Autodesk Fusion 360 part; units mm, degrees
(part 3 of 5)
  spline S405 degree 3 poles (17.0095, -37.7346) (17.0401, -37.6962) (17.0716, -37.6554) (17.1042, -37.6133) knots 24 24 24 24 25 25 25 25
  spline S406 degree 3 poles (17.1042, -37.6133) (17.3273, -37.3244) (17.6051, -36.9649) (17.951, -36.9312) knots 25 25 25 25 26 26 26 26
  spline S407 degree 3 poles (17.951, -36.9312) (18.1537, -36.9124) (18.4001, -37.0615) (18.43, -37.2905) knots 26 26 26 26 27 27 27 27
  ellipse E60 centre (17.4573, -38.1763) end of major axis (17.2727, -40.3787) minor radius 0.995 (18.3658, -38.8335) -> (18.43, -37.2905) ccw
  spline S408 degree 3 poles (18.3658, -38.8335) (18.1975, -39.648) (17.7584, -40.4986) (17.161, -41.1673) knots 28 28 28 28 29 29 29 29
  spline S409 degree 3 poles (9.1607, -35.1495) (9.5148, -36.3147) (10.6476, -37.0396) (11.7092, -37.5945) (11.9284, -37.7091) (12.1669, -37.8283) (12.4344, -37.9569) knots 0 0 0 0 1 1 1 2 2 2 2
  spline S410 degree 3 poles (12.4344, -37.9569) (12.4326, -37.9612) (12.4318, -37.9657) (12.4301, -37.97) knots 2 2 2 2 3 3 3 3
  spline S411 degree 3 poles (12.4301, -37.97) (12.403, -38.0389) (12.3786, -38.1093) (12.3605, -38.1829) knots 3 3 3 3 4 4 4 4
  spline S412 degree 3 poles (12.3605, -38.1829) (12.3365, -38.2818) (12.3232, -38.3821) (12.3214, -38.481) (12.3137, -38.8856) (12.6908, -39.1663) (12.9935, -39.3921) (13.0593, -39.4412) (13.1224, -39.4879) (13.1768, -39.533) knots 4 4 4 4 5 5 5 6 6 6 7 7 7 7
  spline S413 degree 3 poles (13.1768, -39.533) (13.3089, -39.6428) (13.4471, -39.7455) (13.5806, -39.8449) knots 7 7 7 7 8 8 8 8
  line L61 (13.5806, -39.8449) -> (13.6872, -39.9245)
  spline S414 degree 3 poles (13.6872, -39.9245) (14.0165, -40.1718) (14.3068, -40.4614) (14.5874, -40.7415) (14.8134, -40.9671) (15.0471, -41.2003) (15.304, -41.4155) knots 9 9 9 9 10 10 10 11 11 11 11
  spline S415 degree 3 poles (15.304, -41.4155) (15.3519, -41.4555) (15.3989, -41.4971) (15.4457, -41.5385) knots 11 11 11 11 12 12 12 12
  spline S416 degree 3 poles (15.4457, -41.5385) (15.6965, -41.7603) (15.9561, -41.9898) (16.3325, -42.0079) knots 12 12 12 12 13 13 13 13
  spline S417 degree 3 poles (16.3325, -42.0079) (16.3909, -42.0107) (16.4474, -42.0082) (16.5021, -42.0011) (16.5782, -41.9911) (16.6497, -41.9697) (16.7191, -41.9437) (16.7888, -41.9176) (16.8557, -41.8855) (16.9193, -41.8469) (17.1111, -41.7304) (17.2772, -41.5666) (17.4241, -41.4024) knots 13 13 13 13 14 14 14 15 15 15 16 16 16 17 17 17 17
  spline S418 degree 3 poles (17.4241, -41.4024) (17.4279, -41.3981) (17.4313, -41.3935) (17.4351, -41.3892) (17.5055, -41.3099) (17.5736, -41.2281) (17.6397, -41.1443) (17.6657, -41.1113) (17.69, -41.0771) (17.7154, -41.0435) (17.7581, -40.9868) (17.8006, -40.9299) (17.8412, -40.8716) (17.8689, -40.8318) (17.8953, -40.7912) (17.922, -40.7507) knots 17 17 17 17 18 18 18 19 19 19 20 20 20 21 21 21 22 22 22 22
  spline S419 degree 3 poles (17.922, -40.7507) (17.9589, -40.6947) (17.9954, -40.6385) (18.0304, -40.5813) (18.0545, -40.5418) (18.0778, -40.5022) (18.1009, -40.4622) knots 22 22 22 22 23 23 23 24 24 24 24
  spline S420 degree 3 poles (18.1009, -40.4622) (18.1188, -40.4315) (18.1381, -40.4015) (18.1553, -40.3705) knots 24 24 24 24 25 25 25 25
  spline S421 degree 3 poles (18.1553, -40.3705) (18.6984, -40.5996) (19.175, -40.8092) (19.6083, -41.0094) knots 25 25 25 25 26 26 26 26
  spline S422 degree 3 poles (19.6083, -41.0094) (19.9314, -41.2063) (20.2654, -41.4182) (20.629, -41.6572) knots 26 26 26 26 27 27 27 27
  spline S423 degree 3 poles (20.629, -41.6572) (20.7153, -41.7141) (20.8008, -41.7723) (20.8862, -41.8305) knots 27 27 27 27 28 28 28 28
  line L62 (20.8862, -41.8305) -> (21.1231, -41.9905)
  spline S424 degree 3 poles (21.1231, -41.9905) (21.2965, -42.1069) (21.47, -42.2232) (21.6414, -42.3417) (21.7547, -42.4201) (21.8669, -42.4995) (21.9792, -42.579) knots 29 29 29 29 30 30 30 31 31 31 31
  line L63 (21.9792, -42.579) -> (22.2476, -42.7678)
  spline S425 degree 3 poles (22.2476, -42.7678) (22.3833, -42.8629) (22.5192, -42.9581) (22.6541, -43.054) knots 32 32 32 32 33 33 33 33
  line L64 (22.6541, -43.054) -> (23.3329, -43.5393)
  spline S426 degree 3 poles (23.3329, -43.5393) (23.3275, -43.557) (23.3242, -43.5743) (23.3195, -43.5919) knots 34 34 34 34 35 35 35 35
  spline S427 degree 3 poles (23.3195, -43.5919) (23.3148, -43.6089) (23.3104, -43.6257) (23.3065, -43.6426) knots 35 35 35 35 36 36 36 36
  spline S428 degree 3 poles (23.3065, -43.6426) (23.2921, -43.7038) (23.2805, -43.7645) (23.2748, -43.8235) knots 36 36 36 36 37 37 37 37
  spline S429 degree 3 poles (23.2748, -43.8235) (23.2748, -43.8237) (23.2747, -43.8239) (23.2747, -43.824) knots 37 37 37 37 38 38 38 38
  spline S430 degree 3 poles (23.2747, -43.824) (23.253, -44.048) (23.3387, -44.3191) (23.3843, -44.4441) knots 38 38 38 38 39 39 39 39
  ellipse E61 centre (23.3854, -44.4319) end of major axis (23.3496, -44.3317) minor radius 0.0052 (23.3843, -44.4441) -> (23.401, -44.4882) ccw
  spline S431 degree 3 poles (23.401, -44.4882) (23.4621, -44.6444) (23.5572, -44.7939) (23.7005, -44.9589) knots 40 40 40 40 41 41 41 41
  spline S432 degree 3 poles (23.7005, -44.9589) (23.9176, -45.2076) (24.135, -45.3973) (24.3661, -45.5393) knots 41 41 41 41 42 42 42 42
  line L65 (24.3661, -45.5393) -> (24.4057, -45.5638)
  spline S433 degree 3 poles (24.4057, -45.5638) (24.4421, -45.5865) (24.4789, -45.6094) (24.5162, -45.6294) knots 43 43 43 43 44 44 44 44
  arc A9 (24.5162, -45.6294) -> (24.5477, -45.6426) centre (24.6008, -45.4712) ccw
  spline S434 degree 3 poles (24.5477, -45.6426) (24.6194, -45.6647) (24.6914, -45.6848) (24.7636, -45.7029) (24.7855, -45.7084) (24.8076, -45.7126) (24.8296, -45.7178) (24.8802, -45.7297) (24.9309, -45.7417) (24.9818, -45.7516) (25.0059, -45.7563) (25.03, -45.7597) (25.0541, -45.764) (25.1033, -45.7727) (25.1525, -45.7815) (25.2018, -45.7884) (25.2258, -45.7918) (25.2499, -45.794) (25.274, -45.7969) (25.3237, -45.803) (25.3734, -45.8091) (25.4232, -45.8133) (25.4471, -45.8154) (25.471, -45.8163) (25.495, -45.818) (25.545, -45.8213) (25.595, -45.8247) (25.6451, -45.8262) (25.6699, -45.827) (25.6947, -45.8268) (25.7195, -45.8271) (25.7686, -45.8277) (25.8176, -45.8283) (25.8668, -45.8272) (25.8941, -45.8266) (25.9213, -45.825) (25.9486, -45.8238) (25.9947, -45.8219) (26.0408, -45.8199) (26.0869, -45.8165) (26.1189, -45.8141) (26.1509, -45.8106) (26.1829, -45.8075) knots 45 45 45 45 46 46 46 47 47 47 48 48 48 49 49 49 50 50 50 51 51 51 52 52 52 53 53 53 54 54 54 55 55 55 56 56 56 57 57 57 58 58 58 59 59 59 59
  spline S435 degree 3 poles (26.1829, -45.8075) (26.2128, -45.8045) (26.2427, -45.8027) (26.2726, -45.7991) knots 59 59 59 59 60 60 60 60
  spline S436 degree 3 poles (26.2726, -45.7991) (27.1902, -46.394) (27.959, -46.9051) (28.7109, -47.4517) knots 60 60 60 60 61 61 61 61
  line L66 (28.7109, -47.4517) -> (28.9558, -47.6293)
  spline S437 degree 3 poles (28.9558, -47.6293) (29.1234, -47.7506) (29.2998, -47.8781) (29.4804, -48.0117) knots 62 62 62 62 63 63 63 63
  line L67 (29.4804, -48.0117) -> (29.484, -48.0146)
  line L68 (29.484, -48.0146) -> (30.5036, -48.8221)
  line L69 (30.5036, -48.8221) -> (30.5435, -48.8589)
  spline S438 degree 3 poles (30.5435, -48.8589) (30.7296, -49.0293) (31.5071, -49.7424) (32.403, -50.5655) knots 66 66 66 66 67 67 67 67
  spline S439 degree 3 poles (32.403, -50.5655) (32.3945, -50.5754) (32.3858, -50.5865) (32.3773, -50.5966) knots 67 67 67 67 68 68 68 68
  spline S440 degree 3 poles (32.3773, -50.5966) (32.371, -50.6041) (32.3648, -50.6117) (32.3586, -50.6192) knots 68 68 68 68 69 69 69 69
  spline S441 degree 3 poles (32.3586, -50.6192) (32.3317, -50.6517) (32.3053, -50.6846) (32.2797, -50.718) knots 69 69 69 69 70 70 70 70
  spline S442 degree 3 poles (32.2797, -50.718) (32.2765, -50.7221) (32.2735, -50.7263) (32.2703, -50.7305) knots 70 70 70 70 71 71 71 71
  spline S443 degree 3 poles (32.2703, -50.7305) (32.243, -50.7665) (32.2164, -50.8029) (32.1908, -50.8399) knots 71 71 71 71 72 72 72 72
  spline S444 degree 3 poles (32.1908, -50.8399) (32.1886, -50.8431) (32.1865, -50.8465) (32.1842, -50.8497) knots 72 72 72 72 73 73 73 73
  ellipse E62 centre (32.7413, -51.7007) end of major axis (33.3078, -50.2436) minor radius 0.8939 (32.1842, -50.8497) -> (32.0918, -50.9957) ccw
  ellipse E63 centre (37.7927, -51.9009) end of major axis (31.806, -52.0345) minor radius 3.2559 (32.0918, -50.9957) -> (32.0102, -51.1478) ccw
  spline S445 degree 3 poles (32.0102, -51.1478) (31.9954, -51.1779) (31.9808, -51.208) (31.9676, -51.2388) (31.9597, -51.2571) (31.953, -51.2759) (31.9457, -51.2944) (31.9324, -51.3284) (31.9199, -51.3626) (31.9087, -51.3973) knots 75 75 75 75 76 76 76 77 77 77 78 78 78 78
  spline S446 degree 3 poles (31.9087, -51.3973) (31.9028, -51.4156) (31.8973, -51.4341) (31.892, -51.4526) knots 78 78 78 78 79 79 79 79
  spline S447 degree 3 poles (31.892, -51.4526) (31.8812, -51.4905) (31.8719, -51.529) (31.8638, -51.5678) (31.8602, -51.5846) (31.8563, -51.6013) (31.8533, -51.6182) (31.8434, -51.6744) (31.8357, -51.7313) (31.832, -51.7894) (31.8262, -51.8814) (31.8306, -51.9755) (31.8454, -52.0693) knots 79 79 79 79 80 80 80 81 81 81 82 82 82 83 83 83 83
  spline S448 degree 3 poles (31.8454, -52.0693) (31.9055, -52.4449) (32.2971, -52.6397) (32.6118, -52.7963) knots 83 83 83 83 84 84 84 84
  spline S449 degree 3 poles (32.6118, -52.7963) (32.679, -52.8298) (32.7434, -52.8616) (32.7995, -52.8933) (32.9337, -52.9691) (33.072, -53.038) (33.2059, -53.1047) knots 84 84 84 84 85 85 85 86 86 86 86
  line L70 (33.2059, -53.1047) -> (33.3265, -53.165)
  spline S450 degree 3 poles (33.3265, -53.165) (33.6649, -53.3349) (33.9612, -53.5403) (34.2749, -53.7577) (34.5167, -53.9253) (34.7667, -54.0984) (35.0351, -54.2517) knots 87 87 87 87 88 88 88 89 89 89 89
  spline S451 degree 3 poles (35.0351, -54.2517) (35.0845, -54.2801) (35.1336, -54.3099) (35.1825, -54.3397) (35.425, -54.4873) (35.699, -54.6519) (36.0293, -54.6249) knots 89 89 89 89 90 90 90 91 91 91 91
  spline S452 degree 3 poles (36.0293, -54.6249) (36.0435, -54.6237) (36.0573, -54.6244) (36.0717, -54.6225) knots 91 91 91 91 92 92 92 92
  spline S453 degree 3 poles (36.0717, -54.6225) (36.1197, -54.6162) (36.1664, -54.6051) (36.2123, -54.5912) knots 92 92 92 92 93 93 93 93
  spline S454 degree 3 poles (36.2123, -54.5912) (36.2304, -54.5858) (36.2474, -54.5786) (36.2649, -54.5721) knots 93 93 93 93 94 94 94 94
  spline S455 degree 3 poles (36.2649, -54.5721) (36.2903, -54.5626) (36.3154, -54.5527) (36.3395, -54.5412) (36.3627, -54.5302) (36.3849, -54.5178) (36.4069, -54.5051) (36.4231, -54.4957) (36.4391, -54.486) (36.4547, -54.4758) (36.4817, -54.4581) (36.5078, -54.4393) (36.5331, -54.4192) (36.5377, -54.4156) (36.5425, -54.4129) (36.5471, -54.4092) knots 94 94 94 94 95 95 95 96 96 96 97 97 97 98 98 98 99 99 99 99
  spline S456 degree 3 poles (36.5471, -54.4092) (38.0743, -55.8341) (39.6611, -57.2394) (41.1968, -58.5994) (41.594, -58.9511) (41.991, -59.3028) (42.3876, -59.6551) (43.3096, -60.4743) (44.2328, -61.2921) (45.1561, -62.1099) knots 99 99 99 99 100 100 100 101 101 101 102 102 102 102
  line L71 (45.1561, -62.1099) -> (46.4361, -63.2436)
  spline S457 degree 3 poles (46.4361, -63.2436) (46.6035, -63.4107) (46.7725, -63.5762) (46.9415, -63.7418) (47.5199, -64.3084) (48.118, -64.8943) (48.6322, -65.5327) (48.7961, -65.7362) (48.9498, -65.957) (49.0985, -66.1706) (49.2301, -66.3596) (49.3662, -66.5551) (49.5114, -66.7419) (49.5584, -66.8024) (49.6059, -66.8628) (49.6535, -66.9231) knots 103 103 103 103 104 104 104 105 105 105 106 106 106 107 107 107 108 108 108 108
  spline S458 degree 3 poles (49.6535, -66.9231) (49.2873, -66.8806) (48.8648, -66.8491) (48.4098, -66.8491) (47.5059, -66.8491) (46.48, -66.9735) (45.5423, -67.3771) (45.5269, -67.3837) (45.5116, -67.391) (45.4962, -67.3978) (45.4063, -67.4375) (45.3174, -67.48) (45.2294, -67.525) (45.2042, -67.538) (45.1789, -67.5506) (45.1538, -67.564) (45.053, -67.6178) (44.9531, -67.6743) (44.8555, -67.7358) knots 108 108 108 108 109 109 109 110 110 110 111 111 111 112 112 112 113 113 113 114 114 114 114
  spline S459 degree 3 poles (44.8555, -67.7358) (44.844, -67.7431) (44.8329, -67.7513) (44.8215, -67.7587) knots 114 114 114 114 115 115 115 115
  spline S460 degree 3 poles (44.8215, -67.7587) (44.7364, -67.8132) (44.6531, -67.8713) (44.571, -67.9321) (44.5417, -67.9538) (44.5127, -67.9763) (44.4838, -67.9988) (44.457, -68.0197) (44.4294, -68.0391) (44.403, -68.0607) (44.3635, -68.0929) (44.3268, -68.1276) (44.2887, -68.1611) (44.2679, -68.1793) (44.2459, -68.1951) (44.2254, -68.2138) (44.2149, -68.2233) (44.2054, -68.2337) (44.1951, -68.2433) knots 115 115 115 115 116 116 116 117 117 117 118 118 118 119 119 119 120 120 120 121 121 121 121
  spline S461 degree 3 poles (44.1951, -68.2433) (44.1623, -68.2738) (44.131, -68.3055) (44.0993, -68.3369) (44.059, -68.3767) (44.0187, -68.4166) (43.9801, -68.458) (43.9482, -68.4921) (43.9176, -68.5275) (43.8868, -68.5627) (43.8511, -68.6035) (43.8155, -68.6446) (43.7813, -68.6868) (43.7505, -68.7248) (43.7209, -68.7639) (43.6914, -68.803) (43.6598, -68.8448) (43.6285, -68.8868) (43.5984, -68.9299) (43.5691, -68.9717) (43.5408, -69.0145) (43.5129, -69.0575) (43.4852, -69.1002) (43.4579, -69.1432) (43.4314, -69.1871) (43.404, -69.2327) (43.3774, -69.279) (43.3513, -69.3259) (43.327, -69.3696) (43.3033, -69.4138) (43.2802, -69.4587) knots 121 121 121 121 122 122 122 123 123 123 124 124 124 125 125 125 126 126 126 127 127 127 128 128 128 129 129 129 130 130 130 131 131 131 131
  arc A10 (43.2802, -69.4587) -> (43.2065, -69.608) centre (47.6087, -71.6871) ccw
  spline S462 degree 3 poles (43.2065, -69.608) (43.1852, -69.6531) (43.1646, -69.6988) (43.1445, -69.7449) (43.1217, -69.7972) (43.0995, -69.85) (43.0782, -69.9036) (43.0596, -69.9504) (43.042, -69.998) (43.0246, -70.0458) (43.0045, -70.101) (42.9847, -70.1566) (42.9661, -70.2133) knots 132 132 132 132 133 133 133 134 134 134 135 135 135 136 136 136 136
  spline S463 degree 3 poles (42.9661, -70.2133) (42.9502, -70.2619) (42.9353, -70.3115) (42.9205, -70.3611) (42.9032, -70.4191) (42.886, -70.4772) (42.8703, -70.5365) knots 136 136 136 136 137 137 137 138 138 138 138
  spline S464 degree 3 poles (42.8703, -70.5365) (42.8567, -70.5875) (42.8444, -70.6397) (42.832, -70.6917) (42.8177, -70.7519) (42.8033, -70.812) (42.7905, -70.8735) (42.7793, -70.9275) (42.7696, -70.9827) (42.7595, -71.0377) (42.7482, -71.0995) (42.7366, -71.161) (42.7269, -71.2241) (42.7179, -71.282) (42.7106, -71.3414) (42.7029, -71.4004) (42.6947, -71.4629) (42.686, -71.5249) (42.6793, -71.5886) (42.6726, -71.6514) (42.6678, -71.7159) (42.6625, -71.7799) (42.6574, -71.8422) (42.6515, -71.9038) (42.6476, -71.9672) (42.6434, -72.0371) (42.6414, -72.1088) (42.6387, -72.1799) knots 138 138 138 138 139 139 139 140 140 140 141 141 141 142 142 142 143 143 143 144 144 144 145 145 145 146 146 146 147 147 147 147
  spline S465 degree 3 poles (42.6387, -72.1799) (42.6365, -72.2398) (42.6332, -72.2987) (42.6321, -72.3596) (42.6305, -72.443) (42.6315, -72.5286) (42.6321, -72.6138) (42.6324, -72.6647) (42.6315, -72.7144) (42.6326, -72.766) (42.6355, -72.904) (42.6409, -73.0442) (42.6492, -73.1867) knots 147 147 147 147 148 148 148 149 149 149 150 150 150 151 151 151 151
  spline S466 degree 3 poles (42.6492, -73.1867) (42.6534, -73.2587) (42.7009, -73.3208) (42.7691, -73.3438) knots 151 151 151 151 152 152 152 152
  spline S467 degree 3 poles (42.7691, -73.3438) (42.783, -73.3484) (42.8274, -73.363) (42.8976, -73.3839) knots 152 152 152 152 153 153 153 153
  line L72 (42.8976, -73.3839) -> (42.8987, -73.3843)
  spline S468 degree 3 poles (42.8987, -73.3843) (42.9207, -73.3908) (42.9455, -73.3981) (42.9724, -73.4058) (42.9888, -73.4105) (43.0076, -73.4156) (43.0258, -73.4207) (43.0383, -73.4242) (43.0498, -73.4275) (43.0631, -73.4311) (43.0897, -73.4384) (43.1189, -73.4461) (43.1487, -73.4539) (43.1558, -73.4557) (43.1623, -73.4575) (43.1695, -73.4594) knots 154 154 154 154 155 155 155 156 156 156 157 157 157 158 158 158 159 159 159 159
  spline S469 degree 3 poles (43.1695, -73.4594) (43.2046, -73.4684) (43.2421, -73.4778) (43.2811, -73.4874) knots 159 159 159 159 160 160 160 160
  line L73 (43.2811, -73.4874) -> (43.2902, -73.4897)
  spline S470 degree 3 poles (43.2902, -73.4897) (43.3326, -73.5) (43.3774, -73.5106) (43.4242, -73.5213) knots 161 161 161 161 162 162 162 162
  line L74 (43.4242, -73.5213) -> (43.4245, -73.5214)
  spline S471 degree 3 poles (43.4245, -73.5214) (44.4657, -73.76) (46.5503, -74.0551) (48.2956, -73.1753) knots 163 163 163 163 164 164 164 164
  line L75 (48.2956, -73.1753) -> (48.2962, -73.175)
  arc A11 (48.2962, -73.175) -> (48.5289, -73.0493) centre (46.1913, -69.0011) ccw
  spline S472 degree 3 poles (48.5289, -73.0493) (48.5315, -73.0478) (48.534, -73.0463) (48.5365, -73.0448) (48.6109, -73.0016) (48.6846, -72.9562) (48.7574, -72.9083) knots 166 166 166 166 167 167 167 168 168 168 168
  spline S473 degree 3 poles (48.7574, -72.9083) (48.759, -72.9072) (48.7607, -72.9063) (48.7624, -72.9052) knots 168 168 168 168 169 169 169 169
  spline S474 degree 3 poles (48.7624, -72.9052) (48.7659, -72.9029) (48.7691, -72.9003) (48.7726, -72.898) knots 169 169 169 169 170 170 170 170
  spline S475 degree 3 poles (48.7726, -72.898) (48.8213, -72.8656) (48.8703, -72.8341) (48.9181, -72.7996) (48.9366, -72.7863) (48.9535, -72.7713) (48.9717, -72.7577) (48.9923, -72.7423) (49.0121, -72.726) (49.0324, -72.7103) (49.2151, -72.5689) (49.3855, -72.414) (49.5439, -72.2456) (49.561, -72.2273) (49.5786, -72.2094) (49.5955, -72.1908) (49.6425, -72.139) (49.6881, -72.0856) (49.7329, -72.0314) (49.7503, -72.0104) (49.7674, -71.9892) (49.7844, -71.9679) (49.8293, -71.9115) (49.8734, -71.8542) (49.916, -71.7952) knots 170 170 170 170 171 171 171 172 172 172 173 173 173 174 174 174 175 175 175 176 176 176 177 177 177 178 178 178 178
  spline S476 degree 3 poles (49.916, -71.7952) (49.9278, -71.7789) (49.939, -71.7621) (49.9506, -71.7456) knots 178 178 178 178 179 179 179 179
  ellipse E64 centre (-485.3338, 431.1613) end of major axis (-1020.1941, 934.5888) minor radius 58.5616 (49.9506, -71.7456) -> (50.3479, -71.0732) ccw
  spline S477 degree 3 poles (50.3479, -71.0732) (50.3518, -71.0655) (50.3558, -71.058) (50.3596, -71.0503) (50.3952, -70.9771) (50.4288, -70.9019) (50.4618, -70.8259) knots 180 180 180 180 181 181 181 182 182 182 182
  spline S478 degree 3 poles (50.4618, -70.8259) (50.4714, -70.8038) (50.481, -70.7817) (50.4903, -70.7594) (50.5215, -70.685) (50.5514, -70.6095) (50.5801, -70.5324) (50.5884, -70.5099) (50.5964, -70.487) (50.6045, -70.4643) (50.7018, -70.1931) (50.7848, -69.9067) (50.8517, -69.6033) knots 182 182 182 182 183 183 183 184 184 184 185 185 185 186 186 186 186
  spline S479 degree 3 poles (50.8517, -69.6033) (50.8519, -69.6024) (50.8522, -69.6016) (50.8524, -69.6006) knots 186 186 186 186 187 187 187 187
  spline S480 degree 3 poles (50.8524, -69.6006) (50.871, -69.5159) (50.8876, -69.429) (50.9039, -69.3418) (50.9103, -69.3075) (50.917, -69.2733) (50.923, -69.2386) knots 187 187 187 187 188 188 188 189 189 189 189
  spline S481 degree 3 poles (50.923, -69.2386) (50.9374, -69.1559) (50.9506, -69.072) (50.9629, -68.9871) (50.9654, -68.9699) (50.9686, -68.9534) (50.971, -68.936) knots 189 189 189 189 190 190 190 191 191 191 191
  spline S482 degree 3 poles (50.971, -68.936) (51.0928, -69.1731) (51.2187, -69.4158) (51.3517, -69.6359) knots 191 191 191 191 192 192 192 192
  ellipse E65 centre (43.5345, -71.4342) end of major axis (50.5174, -82.0369) minor radius 7.7071 (52.4938, -72.6612) -> (51.3517, -69.6359) ccw
  spline S483 degree 3 poles (52.4938, -72.6612) (49.477, -76.0968) (48.1935, -79.0277) (48.6792, -81.3802) (49.1255, -83.5419) (50.9129, -84.3589) (50.9887, -84.3927) (51.0315, -84.4117) (51.0805, -84.4127) (51.1243, -84.3958) knots 193 193 193 193 194 194 194 195 195 195 196 196 196 196
  spline S484 degree 3 poles (51.1243, -84.3958) (51.2453, -84.3488) (51.3636, -84.2998) (51.4795, -84.2492) (51.5206, -84.2313) (51.5598, -84.2121) (51.6002, -84.1937) (51.6738, -84.1603) (51.7476, -84.1271) (51.819, -84.0922) (51.8665, -84.069) (51.9119, -84.0445) (51.9584, -84.0207) (52.0204, -83.989) (52.0828, -83.9576) (52.143, -83.9247) (52.1918, -83.8981) (52.2387, -83.8702) (52.2864, -83.8429) (52.3417, -83.8111) (52.3975, -83.7797) (52.4514, -83.7469) (52.4999, -83.7174) (52.5467, -83.6867) (52.5941, -83.6563) (52.6444, -83.6241) (52.6951, -83.592) (52.7441, -83.5588) (52.7912, -83.5269) (52.8366, -83.4939) (52.8825, -83.4612) (52.9293, -83.4277) (52.9764, -83.3943) (53.0219, -83.36) (53.0667, -83.3261) (53.1101, -83.2913) (53.1536, -83.2566) (53.1974, -83.2217) (53.2413, -83.1867) (53.2838, -83.1509) (53.3262, -83.1152) (53.3674, -83.0786) (53.4085, -83.042) (53.4496, -83.0054) (53.4907, -82.9687) (53.5305, -82.9312) (53.57, -82.894) (53.6085, -82.8561) (53.6467, -82.818) (53.6856, -82.7793) (53.7242, -82.7404) (53.7618, -82.7008) knots 196 196 196 196 197 197 197 198 198 198 199 199 199 200 200 200 201 201 201 202 202 202 203 203 203 204 204 204 205 205 205 206 206 206 207 207 207 208 208 208 209 209 209 210 210 210 211 211 211 212 212 212 213 213 213 213
  spline S485 degree 3 poles (53.7618, -82.7008) (53.7982, -82.6624) (53.8338, -82.6233) (53.869, -82.5841) knots 213 213 213 213 214 214 214 214
  spline S486 degree 3 poles (53.869, -82.5841) (53.9058, -82.5431) (53.942, -82.5018) (53.9773, -82.4599) (54.0107, -82.4204) (54.0434, -82.3804) (54.0755, -82.3401) (54.1102, -82.2966) (54.1441, -82.2527) (54.1773, -82.2083) (54.2075, -82.168) (54.2371, -82.1273) (54.2662, -82.0862) knots 214 214 214 214 215 215 215 216 216 216 217 217 217 218 218 218 218
  spline S487 degree 3 poles (54.2662, -82.0862) (54.2987, -82.04) (54.3304, -81.9931) (54.3615, -81.9459) (54.3884, -81.9051) (54.4151, -81.864) (54.4409, -81.8224) (54.4714, -81.773) (54.5008, -81.723) (54.5298, -81.6726) (54.5535, -81.6314) (54.5772, -81.5903) (54.5998, -81.5484) (54.6281, -81.4959) (54.6551, -81.4425) (54.6818, -81.389) knots 218 218 218 218 219 219 219 220 220 220 221 221 221 222 222 222 223 223 223 223
  spline S488 degree 3 poles (54.6818, -81.389) (54.7025, -81.3474) (54.7234, -81.306) (54.743, -81.2638) (54.7689, -81.2084) (54.7931, -81.152) (54.8172, -81.0955) (54.8352, -81.0534) (54.8534, -81.0115) (54.8704, -80.9688) (54.8763, -80.9541) (54.883, -80.94) (54.8888, -80.9252) (54.9113, -80.8671) (54.9312, -80.8084) (54.9518, -80.7498) (54.9582, -80.7315) (54.9657, -80.7138) (54.972, -80.6954) knots 223 223 223 223 224 224 224 225 225 225 226 226 226 227 227 227 228 228 228 229 229 229 229
  spline S489 degree 3 poles (54.972, -80.6954) (54.9733, -80.6915) (54.9743, -80.6875) (54.9756, -80.6835) knots 229 229 229 229 230 230 230 230
  arc A12 (54.9756, -80.6835) -> (55.0773, -80.3483) centre (49.3167, -78.7838) ccw
  spline S490 degree 3 poles (55.0773, -80.3483) (55.0809, -80.3349) (55.084, -80.3214) (55.0876, -80.308) knots 231 231 231 231 232 232 232 232
  spline S491 degree 3 poles (55.0876, -80.308) (55.1143, -80.2067) (55.1384, -80.105) (55.16, -80.0029) (55.1638, -79.985) (55.1676, -79.9671) (55.1712, -79.9492) knots 232 232 232 232 233 233 233 234 234 234 234
  ellipse E66 centre (24.4608, -64.2546) end of major axis (-5.574, -46.7642) minor radius 13.9771 (55.1712, -79.9492) -> (55.3003, -78.8826) ccw
  line L76 (55.3003, -78.8826) -> (55.301, -78.8667)
  ellipse E67 centre (37.5646, -70.719) end of major axis (20.8518, -59.3182) minor radius 10.5763 (55.301, -78.8667) -> (55.2771, -77.7932) ccw
  spline S492 degree 3 poles (55.2771, -77.7932) (55.2758, -77.7777) (55.2744, -77.7621) (55.273, -77.7466) (55.2641, -77.6466) (55.2536, -77.547) (55.2417, -77.4478) (55.2395, -77.429) (55.2375, -77.4101) (55.2352, -77.3914) knots 237 237 237 237 238 238 238 239 239 239 240 240 240 240
  spline S493 degree 3 poles (55.2352, -77.3914) (55.2216, -77.2828) (55.2063, -77.1748) (55.1894, -77.0674) (55.1833, -77.0284) (55.1762, -76.9898) (55.1696, -76.951) (55.1593, -76.89) (55.1488, -76.8292) (55.1376, -76.7687) (55.1254, -76.7034) (55.1126, -76.6386) (55.0995, -76.5739) (55.0944, -76.5491) (55.0892, -76.5244) (55.084, -76.4997) knots 240 240 240 240 241 241 241 242 242 242 243 243 243 244 244 244 245 245 245 245
  spline S494 degree 3 poles (55.084, -76.4997) (54.7762, -75.0337) (54.2156, -73.7332) (53.8123, -72.9225) knots 245 245 245 245 246 246 246 246
  ellipse E68 centre (48.0724, -66.8569) end of major axis (44.1035, -56.4654) minor radius 4.4389 (53.8123, -72.9225) -> (53.7916, -72.1467) ccw
  spline S495 degree 3 poles (53.7916, -72.1467) (54.1354, -72.7806) (54.5781, -73.438) (55.1292, -73.9842) knots 247 247 247 247 248 248 248 248
  spline S496 degree 3 poles (55.1292, -73.9842) (55.1337, -73.9886) (55.1382, -73.9931) (55.1426, -73.9975) (55.2006, -74.0546) (55.2599, -74.1101) (55.3202, -74.1645) (55.3349, -74.1777) (55.3493, -74.1911) (55.3641, -74.2041) knots 248 248 248 248 249 249 249 250 250 250 251 251 251 251
  spline S497 degree 3 poles (55.3641, -74.2041) (55.4151, -74.249) (55.4672, -74.2925) (55.5199, -74.3353) (55.5435, -74.3545) (55.5669, -74.3741) (55.5909, -74.3929) (55.6362, -74.4282) (55.6825, -74.462) (55.7289, -74.4957) (55.7605, -74.5186) (55.7918, -74.5419) (55.824, -74.564) (55.8646, -74.5919) (55.9064, -74.6181) (55.9479, -74.6446) (55.9865, -74.6691) (56.0246, -74.6942) (56.0639, -74.7176) (56.1013, -74.7397) (56.1398, -74.76) (56.1779, -74.7809) (56.2223, -74.8054) (56.2663, -74.8305) (56.3117, -74.8532) (56.3476, -74.8712) (56.3847, -74.8871) (56.4213, -74.904) (56.4698, -74.9265) (56.5178, -74.9498) (56.5675, -74.9703) (56.6066, -74.9864) (56.6472, -75) (56.687, -75.0149) (56.7351, -75.0328) (56.7826, -75.0519) (56.8318, -75.0679) knots 251 251 251 251 252 252 252 253 253 253 254 254 254 255 255 255 256 256 256 257 257 257 258 258 258 259 259 259 260 260 260 261 261 261 262 262 262 263 263 263 263
  spline S498 degree 3 poles (56.8318, -75.0679) (56.8333, -75.0684) (56.8347, -75.0691) (56.8363, -75.0696) knots 263 263 263 263 264 264 264 264
  spline S499 degree 3 poles (56.8363, -75.0696) (56.9029, -75.0912) (56.9702, -75.1087) (57.0375, -75.1263) knots 264 264 264 264 265 265 265 265
  spline S500 degree 3 poles (57.0375, -75.1263) (57.0601, -75.1321) (57.0818, -75.1398) (57.1045, -75.1452) knots 265 265 265 265 266 266 266 266
  line L77 (57.1045, -75.1452) -> (57.0886, -75.142)
  spline S501 degree 3 poles (57.0886, -75.142) (57.1061, -75.1462) (57.1239, -75.1487) (57.1415, -75.1527) (57.212, -75.1684) (57.2826, -75.1832) (57.3538, -75.1946) (57.3955, -75.2012) (57.4377, -75.205) (57.4796, -75.2101) (57.527, -75.2159) (57.5743, -75.2226) (57.6221, -75.2265) (57.6705, -75.2305) (57.7193, -75.2316) (57.768, -75.2336) (57.8099, -75.2353) (57.8517, -75.2378) (57.8939, -75.238) (57.9455, -75.2383) (57.9976, -75.236) (58.0496, -75.2341) (58.0894, -75.2327) (58.1291, -75.2318) (58.1691, -75.2291) (58.2229, -75.2254) (58.277, -75.2194) (58.3312, -75.2134) (58.3699, -75.2091) (58.4087, -75.2051) (58.4477, -75.1997) (58.5029, -75.1919) (58.5585, -75.1821) (58.6141, -75.172) (58.6526, -75.165) (58.6911, -75.1579) (58.7299, -75.1498) (58.7862, -75.1379) (58.8428, -75.1243) (58.8995, -75.11) (58.9381, -75.1002) (58.9767, -75.0902) (59.0155, -75.0794) (59.0724, -75.0634) (59.1295, -75.0461) (59.1869, -75.0278) (59.2263, -75.0151) (59.2658, -75.0019) (59.3054, -74.9881) (59.3623, -74.9683) (59.4195, -74.9475) (59.4767, -74.9253) (59.5174, -74.9096) (59.5583, -74.8929) (59.5992, -74.876) (59.6559, -74.8525) (59.7128, -74.8283) (59.7699, -74.8025) (59.8121, -74.7834) (59.8545, -74.7631) (59.8969, -74.7427) (59.953, -74.7158) (60.0092, -74.6886) (60.0657, -74.6595) (60.1102, -74.6365) (60.155, -74.6119) (60.1998, -74.5875) (60.2546, -74.5577) (60.3093, -74.5281) (60.3644, -74.4962) (60.4124, -74.4685) (60.4607, -74.4387) (60.5089, -74.4094) (60.5613, -74.3775) (60.6136, -74.3463) (60.6663, -74.3126) (60.7192, -74.2787) (60.7725, -74.2424) (60.8256, -74.2066) (60.8742, -74.174) (60.9227, -74.1424) (60.9715, -74.1082) (61.0339, -74.0645) (61.0966, -74.0179) (61.1593, -73.9717) (61.1995, -73.942) (61.2396, -73.9139) (61.28, -73.8832) (61.3835, -73.8045) (61.4874, -73.7228) (61.5919, -73.6373) (61.6301, -73.6059) (61.6529, -73.5606) (61.6561, -73.5128) (61.6572, -73.4968) (61.6562, -73.4805) (61.6528, -73.4644) knots 267 267 267 267 268 268 268 269 269 269 270 270 270 271 271 271 272 272 272 273 273 273 274 274 274 275 275 275 276 276 276 277 277 277 278 278 278 279 279 279 280 280 280 281 281 281 282 282 282 283 283 283 284 284 284 285 285 285 286 286 286 287 287 287 288 288 288 289 289 289 290 290 290 291 291 291 292 292 292 293 293 293 294 294 294 295 295 295 296 296 296 297 297 297 298 298 298 299 299 299 299
  spline S502 degree 3 poles (61.6528, -73.4644) (61.6517, -73.4595) (61.6491, -73.4476) (61.6454, -73.4317) knots 299 299 299 299 300 300 300 300
  spline S503 degree 3 poles (61.6454, -73.4317) (61.5771, -73.1385) (61.0291, -71.0534) (59.0331, -69.8622) (58.134, -69.3257) (57.0851, -69.0573) (55.8967, -69.0574) (55.119, -69.0575) (54.2811, -69.1737) (53.3867, -69.404) knots 300 300 300 300 301 301 301 302 302 302 303 303 303 303
  ellipse E69 centre (35.8916, -66.1831) end of major axis (20.5604, -52.0655) minor radius 13.7082 (53.3867, -69.404) -> (51.9599, -65.262) ccw
  spline S504 degree 3 poles (51.9599, -65.262) (53.2122, -65.7163) (54.5148, -65.9538) (55.6442, -66.1266) (56.138, -66.2022) (56.6543, -66.2661) (57.1538, -66.3279) (59.1045, -66.5694) (61.1217, -66.8191) (62.7538, -67.8227) knots 304 304 304 304 305 305 305 306 306 306 307 307 307 307
  spline S505 degree 3 poles (62.7538, -67.8227) (62.9133, -67.9429) (63.1017, -68.0812) (63.301, -68.2076) knots 307 307 307 307 308 308 308 308
  spline S506 degree 3 poles (63.301, -68.2076) (62.8168, -69.1853) (62.139, -71.0646) (62.6864, -73.1703) (62.7066, -73.2481) (62.7277, -73.326) (62.7514, -73.4044) (62.7584, -73.4278) (62.7665, -73.4513) (62.7739, -73.4747) knots 308 308 308 308 309 309 309 310 310 310 311 311 311 311
  spline S507 degree 3 poles (62.7739, -73.4747) (62.7967, -73.5469) (62.8205, -73.6191) (62.8463, -73.6917) (62.85, -73.702) (62.8529, -73.7122) (62.8566, -73.7226) knots 311 311 311 311 312 312 312 313 313 313 313
  spline S508 degree 3 poles (62.8566, -73.7226) (62.8622, -73.738) (62.8687, -73.7531) (62.8744, -73.7685) knots 313 313 313 313 314 314 314 314
  spline S509 degree 3 poles (62.8744, -73.7685) (62.8968, -73.8291) (62.9202, -73.8895) (62.9445, -73.9495) (62.9553, -73.9763) (62.9663, -74.003) (62.9775, -74.0296) (62.9868, -74.0518) (62.9952, -74.074) (63.0049, -74.0963) (63.0182, -74.1268) (63.033, -74.1568) (63.0468, -74.1871) knots 314 314 314 314 315 315 315 316 316 316 317 317 317 318 318 318 318
  spline S510 degree 3 poles (63.0468, -74.1871) (63.0643, -74.2259) (63.0819, -74.2647) (63.1003, -74.3032) (63.1206, -74.3459) (63.1419, -74.3883) (63.1632, -74.4306) knots 318 318 318 318 319 319 319 320 320 320 320
  spline S511 degree 3 poles (63.1632, -74.4306) (63.1861, -74.4762) (63.2091, -74.5218) (63.2332, -74.567) (63.2511, -74.6007) (63.27, -74.6341) (63.2885, -74.6677) knots 320 320 320 320 321 321 321 322 322 322 322
  spline S512 degree 3 poles (63.2885, -74.6677) (63.3177, -74.7203) (63.347, -74.7729) (63.3778, -74.8251) knots 322 322 322 322 323 323 323 323
  spline S513 degree 3 poles (63.3778, -74.8251) (63.3919, -74.8491) (63.4069, -74.8729) (63.4214, -74.8968) knots 323 323 323 323 324 324 324 324
  spline S514 degree 3 poles (63.4214, -74.8968) (63.4582, -74.9575) (63.4953, -75.018) (63.5342, -75.078) knots 324 324 324 324 325 325 325 325
  spline S515 degree 3 poles (63.5342, -75.078) (63.5424, -75.0906) (63.551, -75.103) (63.5592, -75.1155) knots 325 325 325 325 326 326 326 326
  ellipse E70 centre (232.856, -19.216) end of major axis (63.0285, -73.9056) minor radius 33.8867 (63.5592, -75.1155) -> (70.1202, -79.9149) ccw
  spline S516 degree 3 poles (70.1202, -79.9149) (70.1237, -79.9167) (70.1272, -79.9185) (70.1307, -79.9204) knots 327 327 327 327 328 328 328 328
  spline S517 degree 3 poles (70.1307, -79.9204) (70.2318, -79.9735) (70.3347, -80.026) (70.439, -80.0779) (70.4481, -80.0824) (70.4572, -80.087) (70.4663, -80.0915) knots 328 328 328 328 329 329 329 330 330 330 330
  spline S518 degree 3 poles (70.4663, -80.0915) (70.5646, -80.1446) (70.6644, -80.1971) (70.7656, -80.2491) (70.7795, -80.2562) (70.7934, -80.2633) (70.8074, -80.2704) (70.9045, -80.3199) (71.0028, -80.3689) (71.1026, -80.4174) (71.1225, -80.427) (71.1424, -80.4367) (71.1624, -80.4463) (71.2582, -80.4924) (71.355, -80.538) (71.4532, -80.5832) (71.4782, -80.5946) (71.5033, -80.606) (71.5284, -80.6175) (71.6231, -80.6605) (71.7187, -80.7032) (71.8156, -80.7453) (71.8462, -80.7587) (71.8771, -80.7719) (71.9079, -80.7851) (72.0011, -80.8251) (72.095, -80.8648) (72.1902, -80.904) (72.2266, -80.919) (72.2635, -80.9338) (72.3002, -80.9487) (72.3916, -80.9858) (72.4835, -81.0227) (72.5768, -81.059) (72.6196, -81.0757) (72.663, -81.0921) (72.7062, -81.1087) (72.7954, -81.1428) (72.8847, -81.1768) (72.9756, -81.2103) (73.0253, -81.2287) (73.076, -81.2467) (73.1262, -81.2649) (73.2125, -81.2961) (73.2988, -81.3272) (73.3866, -81.3579) (73.444, -81.3779) (73.5026, -81.3975) (73.5606, -81.4173) (73.6434, -81.4456) (73.7259, -81.4739) (73.8099, -81.5016) (73.8763, -81.5235) (73.944, -81.5449) (74.0111, -81.5665) (74.089, -81.5916) (74.1665, -81.6168) (74.2455, -81.6415) (74.3225, -81.6655) (74.4009, -81.6889) (74.4789, -81.7125) (74.5507, -81.7342) (74.6217, -81.7562) (74.6943, -81.7776) (74.7887, -81.8054) (74.8849, -81.8325) (74.9807, -81.8598) (75.0387, -81.8763) (75.0958, -81.8932) (75.1543, -81.9094) (75.3103, -81.9529) (75.468, -81.9956) (75.6278, -82.0375) knots 330 330 330 330 331 331 331 332 332 332 333 333 333 334 334 334 335 335 335 336 336 336 337 337 337 338 338 338 339 339 339 340 340 340 341 341 341 342 342 342 343 343 343 344 344 344 345 345 345 346 346 346 347 347 347 348 348 348 349 349 349 350 350 350 351 351 351 352 352 352 353 353 353 354 354 354 354
  spline S519 degree 3 poles (75.6278, -82.0375) (75.7152, -82.0579) (75.8006, -82.0123) (75.8331, -81.9307) knots 354 354 354 354 355 355 355 355
  spline S520 degree 3 poles (75.8331, -81.9307) (75.8476, -81.895) (75.923, -81.706) (76.0211, -81.3991) (76.0255, -81.3852) (76.0303, -81.3693) (76.0348, -81.355) knots 355 355 355 355 356 356 356 357 357 357 357
  spline S521 degree 3 poles (76.0348, -81.355) (76.0464, -81.3172) (76.0579, -81.2794) (76.07, -81.2383) knots 357 357 357 357 358 358 358 358
  spline S522 degree 3 poles (76.07, -81.2383) (76.08, -81.2044) (76.0903, -81.1673) (76.1005, -81.1313) knots 358 358 358 358 359 359 359 359
  spline S523 degree 3 poles (76.1005, -81.1313) (76.1076, -81.1068) (76.1146, -81.0838) (76.1218, -81.0585) (76.1362, -81.0079) (76.1508, -80.9541) (76.1654, -80.8998) (76.1689, -80.8869) (76.1724, -80.875) (76.1759, -80.8618) knots 359 359 359 359 360 360 360 361 361 361 362 362 362 362
  spline S524 degree 3 poles (76.1759, -80.8618) (76.1927, -80.7983) (76.2096, -80.7318) (76.2265, -80.6637) knots 362 362 362 362 363 363 363 363
  spline S525 degree 3 poles (76.2265, -80.6637) (76.2278, -80.6583) (76.2291, -80.6533) (76.2304, -80.6479) knots 363 363 363 363 364 364 364 364
  spline S526 degree 3 poles (76.2304, -80.6479) (76.5967, -79.8064) (77.0162, -78.5914) (77.1512, -77.2229) knots 364 364 364 364 365 365 365 365
  line L78 (77.1512, -77.2229) -> (72.1257, -81.7777)
  spline S527 degree 3 poles (72.1257, -81.7777) (72.1385, -81.6653) (72.1492, -81.5519) (72.1581, -81.4374) knots 366 366 366 366 367 367 367 367
  line L79 (72.1581, -81.4374) -> (72.6686, -75.3073)
  spline S528 degree 3 poles (72.6686, -75.3073) (72.6626, -75.1952) (72.6542, -75.0825) (72.6438, -74.9692) knots 368 368 368 368 369 369 369 369
  spline S529 degree 3 poles (72.6438, -74.9692) (72.6434, -74.9647) (72.6432, -74.9603) (72.6427, -74.9558) knots 369 369 369 369 370 370 370 370
  spline S530 degree 3 poles (72.6427, -74.9558) (72.6323, -74.8448) (72.6193, -74.7334) (72.6044, -74.6216) knots 370 370 370 370 371 371 371 371
  spline S531 degree 3 poles (72.6044, -74.6216) (72.6035, -74.6147) (72.6028, -74.608) (72.6018, -74.6012) knots 371 371 371 371 372 372 372 372
  spline S532 degree 3 poles (72.6018, -74.6012) (72.5869, -74.4921) (72.5692, -74.3828) (72.5497, -74.2732) knots 372 372 372 372 373 373 373 373
  spline S533 degree 3 poles (72.5497, -74.2732) (72.5479, -74.2634) (72.5465, -74.2536) (72.5447, -74.2438) knots 373 373 373 373 374 374 374 374
  spline S534 degree 3 poles (72.5447, -74.2438) (72.5251, -74.1369) (72.5027, -74.0297) (72.4784, -73.9225) knots 374 374 374 374 375 375 375 375
  spline S535 degree 3 poles (72.4784, -73.9225) (72.4757, -73.91) (72.4734, -73.8976) (72.4706, -73.8852) (72.4466, -73.7803) (72.4197, -73.6753) (72.391, -73.5703) (72.3869, -73.5555) (72.3835, -73.5406) (72.3793, -73.5258) (72.3508, -73.424) (72.3191, -73.3223) (72.2859, -73.2207) (72.2799, -73.2025) (72.2747, -73.1842) (72.2686, -73.1661) knots 375 375 375 375 376 376 376 377 377 377 378 378 378 379 379 379 380 380 380 380
  spline S536 degree 3 poles (72.2686, -73.1661) (72.2351, -73.0678) (72.1985, -72.9698) (72.1603, -72.8719) (72.1521, -72.8507) (72.1446, -72.8293) (72.1361, -72.8081) knots 380 380 380 380 381 381 381 382 382 382 382
  spline S537 degree 3 poles (72.1361, -72.8081) (72.0984, -72.7134) (72.0573, -72.619) (72.015, -72.5248) (72.0041, -72.5006) (71.9941, -72.4762) (71.9829, -72.452) (71.9407, -72.361) (71.8951, -72.2706) (71.8484, -72.1803) (71.8372, -72.1587) (71.8276, -72.1369) (71.8162, -72.1153) (71.8137, -72.1106) (71.8107, -72.1062) (71.8082, -72.1015) knots 382 382 382 382 383 383 383 384 384 384 385 385 385 386 386 386 387 387 387 387
  spline S538 degree 3 poles (71.8082, -72.1015) (71.7982, -72.0812) (71.7898, -72.0608) (71.7796, -72.0406) (71.7401, -71.9624) (71.6948, -71.8876) (71.6524, -71.8111) (71.6204, -71.7533) (71.59, -71.6946) (71.5564, -71.6377) (71.503, -71.5475) (71.445, -71.4599) (71.3874, -71.3721) (71.3506, -71.3159) (71.3149, -71.259) (71.2764, -71.2038) (71.2161, -71.1176) (71.1518, -71.0338) (71.0874, -70.9501) (71.0464, -70.8967) (71.0061, -70.8427) (70.9634, -70.7903) (70.896, -70.7077) (70.8249, -70.6274) (70.7534, -70.5473) (70.7084, -70.497) (70.664, -70.4463) (70.6174, -70.397) (70.5428, -70.318) (70.4648, -70.2411) (70.3861, -70.1647) (70.3373, -70.1174) (70.2887, -70.0699) (70.2384, -70.0236) (70.1565, -69.9483) (70.0715, -69.8749) (69.9854, -69.8021) (69.9331, -69.7579) (69.8807, -69.7138) (69.8268, -69.6706) (69.7374, -69.5989) (69.6453, -69.5289) (69.5516, -69.4598) (69.4958, -69.4187) (69.4397, -69.3778) (69.3824, -69.3376) (69.2856, -69.2697) (69.1864, -69.2033) (69.0853, -69.1381) (69.026, -69.0998) (68.9661, -69.062) (68.9052, -69.0246) (68.8012, -68.9607) (68.695, -68.898) (68.5865, -68.8368) (68.5236, -68.8013) (68.4598, -68.7664) (68.3954, -68.7318) (68.284, -68.6719) (68.1709, -68.613) (68.0552, -68.5559) (67.9887, -68.5231) (67.921, -68.4911) (67.8531, -68.4591) (67.7346, -68.4034) (67.6146, -68.3485) (67.4917, -68.2955) (67.4215, -68.2653) (67.3497, -68.236) (67.278, -68.2066) (67.1524, -68.1551) (67.0256, -68.1043) (66.8956, -68.0555) (66.822, -68.0279) (66.7464, -68.0015) (66.6714, -67.9748) (66.5384, -67.9274) (66.4045, -67.8805) (66.267, -67.8359) (66.1903, -67.811) (66.1115, -67.7876) (66.0334, -67.7636) (65.8926, -67.7203) (65.7514, -67.6773) (65.6061, -67.6368) (65.5268, -67.6148) (65.4451, -67.5942) (65.3645, -67.573) (65.2155, -67.5338) (65.0663, -67.4946) (64.9128, -67.4583) (64.8327, -67.4393) (64.7499, -67.4221) (64.6686, -67.4039) (64.5093, -67.3683) (64.3499, -67.3327) (64.1859, -67.3001) (64.1734, -67.2977) (64.1616, -67.2947) (64.1491, -67.2922) knots 387 387 387 387 388 388 388 389 389 389 390 390 390 391 391 391 392 392 392 393 393 393 394 394 394 395 395 395 396 396 396 397 397 397 398 398 398 399 399 399 400 400 400 401 401 401 402 402 402 403 403 403 404 404 404 405 405 405 406 406 406 407 407 407 408 408 408 409 409 409 410 410 410 411 411 411 412 412 412 413 413 413 414 414 414 415 415 415 416 416 416 417 417 417 418 418 418 419 419 419 420 420 420 420
  ellipse E71 centre (63.6319, -67.5937) end of major axis (63.4657, -67.4063) minor radius 0.665 (64.1491, -67.2922) -> (64.1532, -67.2719) ccw
  spline S539 degree 3 poles (64.1532, -67.2719) (65.4461, -67.3339) (67.2153, -67.1906) (68.5802, -66.2273) knots 421 421 421 421 422 422 422 422
  spline S540 degree 3 poles (68.5802, -66.2273) (68.5943, -66.2172) (68.6085, -66.2071) (68.6226, -66.1968) knots 422 422 422 422 423 423 423 423
  spline S541 degree 3 poles (68.6226, -66.1968) (68.7, -66.1401) (68.7759, -66.0807) (68.8504, -66.0185) (68.8685, -66.0034) (68.8871, -65.9892) (68.905, -65.9737) knots 423 423 423 423 424 424 424 425 425 425 425
  spline S542 degree 3 poles (68.905, -65.9737) (68.9138, -65.9661) (68.923, -65.9594) (68.9318, -65.9518) (69.0114, -65.882) (69.0881, -65.8095) (69.162, -65.7347) knots 425 425 425 425 426 426 426 427 427 427 427
  spline S543 degree 3 poles (69.162, -65.7347) (69.1626, -65.734) (69.1633, -65.7334) (69.164, -65.7328) knots 427 427 427 427 428 428 428 428
  spline S544 degree 3 poles (69.164, -65.7328) (69.2349, -65.6627) (69.303, -65.5902) (69.3688, -65.5156) (69.3915, -65.4897) (69.4123, -65.4622) (69.4345, -65.4359) (69.4769, -65.3853) (69.5194, -65.335) (69.5596, -65.2825) (69.5868, -65.2467) (69.6121, -65.2092) (69.6383, -65.1725) (69.6707, -65.1272) (69.7035, -65.0823) (69.7342, -65.0356) (69.7615, -64.9942) (69.7869, -64.9511) (69.813, -64.9086) (69.84, -64.8644) (69.8673, -64.8206) (69.893, -64.7752) (69.9188, -64.7295) (69.943, -64.6823) (69.9675, -64.6353) (69.9907, -64.5908) (70.0141, -64.5464) (70.036, -64.5008) (70.0597, -64.4516) (70.082, -64.4011) (70.1042, -64.3506) (70.1243, -64.305) (70.1444, -64.2592) (70.1633, -64.2125) (70.1844, -64.1602) (70.2044, -64.1069) (70.2241, -64.0533) (70.2414, -64.006) (70.2585, -63.9585) (70.2746, -63.9102) (70.293, -63.8553) (70.3106, -63.7995) (70.3275, -63.7433) (70.3423, -63.694) (70.3566, -63.6442) (70.3702, -63.5939) (70.3858, -63.5366) (70.4006, -63.4788) (70.4146, -63.4203) knots 428 428 428 428 429 429 429 430 430 430 431 431 431 432 432 432 433 433 433 434 434 434 435 435 435 436 436 436 437 437 437 438 438 438 439 439 439 440 440 440 441 441 441 442 442 442 443 443 443 444 444 444 444
  spline S545 degree 3 poles (70.4146, -63.4203) (70.4265, -63.3682) (70.4374, -63.3154) (70.448, -63.2623) (70.4598, -63.2033) (70.4711, -63.144) (70.4814, -63.0837) (70.4908, -63.0282) (70.4992, -62.9718) (70.5074, -62.9152) knots 444 444 444 444 445 445 445 446 446 446 447 447 447 447
  spline S546 degree 3 poles (70.5074, -62.9152) (70.5168, -62.8553) (70.5262, -62.7954) (70.5342, -62.7343) (70.542, -62.6748) (70.5484, -62.6142) (70.5549, -62.5535) (70.5613, -62.4932) (70.568, -62.4331) (70.5731, -62.3717) (70.5784, -62.3071) (70.5821, -62.241) (70.586, -62.1752) (70.5895, -62.1156) (70.5936, -62.0564) (70.5959, -61.9958) (70.5986, -61.9236) (70.5994, -61.8498) (70.6004, -61.7762) (70.6012, -61.7196) (70.603, -61.6638) (70.6028, -61.6064) (70.6024, -61.5207) (70.5997, -61.433) (70.5971, -61.3455) (70.5957, -61.2979) (70.5956, -61.2514) (70.5935, -61.2033) (70.5876, -61.0663) (70.5793, -60.9274) (70.568, -60.786) knots 447 447 447 447 448 448 448 449 449 449 450 450 450 451 451 451 452 452 452 453 453 453 454 454 454 455 455 455 456 456 456 457 457 457 457
  spline S547 degree 3 poles (70.568, -60.786) (70.5612, -60.7143) (70.5114, -60.6539) (70.4424, -60.6336) knots 457 457 457 457 458 458 458 458
  spline S548 degree 3 poles (70.4424, -60.6336) (70.434, -60.6311) (70.4131, -60.6252) (70.3848, -60.6174) knots 458 458 458 458 459 459 459 459
  spline S549 degree 3 poles (70.3848, -60.6174) (70.3816, -60.6165) (70.3794, -60.6159) (70.3759, -60.615) knots 459 459 459 459 460 460 460 460
  spline S550 degree 3 poles (70.3759, -60.615) (70.364, -60.6117) (70.3492, -60.6079) (70.3343, -60.604) (70.3272, -60.6021) (70.3209, -60.6004) (70.3132, -60.5984) (70.2978, -60.5944) (70.2802, -60.59) (70.2624, -60.5856) knots 460 460 460 460 461 461 461 462 462 462 463 463 463 463
  spline S551 degree 3 poles (70.2624, -60.5856) (70.2526, -60.5831) (70.2433, -60.5808) (70.2327, -60.5782) (70.2133, -60.5734) (70.1919, -60.5684) (70.1701, -60.5632) (70.1589, -60.5606) (70.1481, -60.558) (70.1363, -60.5552) knots 463 463 463 463 464 464 464 465 465 465 466 466 466 466
  spline S552 degree 3 poles (70.1363, -60.5552) (70.1127, -60.5498) (70.0875, -60.5441) (70.0616, -60.5383) (70.049, -60.5355) (70.0365, -60.5327) (70.0234, -60.5298) (69.9962, -60.5239) (69.9677, -60.5179) (69.9384, -60.5118) (69.9241, -60.5088) (69.9097, -60.5058) (69.8948, -60.5028) (69.8644, -60.4966) (69.8329, -60.4904) (69.8003, -60.4842) (69.7846, -60.4811) (69.7687, -60.4781) (69.7525, -60.4751) (69.7187, -60.4687) (69.684, -60.4625) (69.6482, -60.4561) knots 466 466 466 466 467 467 467 468 468 468 469 469 469 470 470 470 471 471 471 472 472 472 473 473 473 473
  spline S553 degree 3 poles (69.6482, -60.4561) (69.6313, -60.4531) (69.6141, -60.4501) (69.5967, -60.4471) (69.5598, -60.4406) (69.5222, -60.4343) (69.4833, -60.428) (69.4654, -60.4251) (69.447, -60.4222) (69.4287, -60.4194) (69.3885, -60.4131) (69.3477, -60.4069) (69.3057, -60.4008) (69.2877, -60.3982) (69.2691, -60.3957) (69.2508, -60.3932) (69.2067, -60.3871) (69.1623, -60.3811) (69.1164, -60.3754) (69.099, -60.3732) (69.081, -60.3712) (69.0634, -60.3691) (69.0154, -60.3633) (68.9671, -60.3578) (68.9173, -60.3526) (68.9015, -60.3509) (68.8851, -60.3494) (68.8691, -60.3478) (68.816, -60.3425) (68.7625, -60.3375) (68.7075, -60.3329) (68.697, -60.332) (68.6861, -60.3313) (68.6755, -60.3305) (68.4759, -60.3146) (68.2662, -60.3035) (68.0477, -60.301) (67.6656, -60.2965) (67.2594, -60.3172) (66.8464, -60.3759) knots 473 473 473 473 474 474 474 475 475 475 476 476 476 477 477 477 478 478 478 479 479 479 480 480 480 481 481 481 482 482 482 483 483 483 484 484 484 485 485 485 486 486 486 486
  spline S554 degree 3 poles (66.8464, -60.3759) (66.8445, -60.3762) (66.8426, -60.3766) (66.8407, -60.3768) knots 486 486 486 486 487 487 487 487
  spline S555 degree 3 poles (66.8407, -60.3768) (66.7614, -60.3886) (66.6819, -60.4018) (66.6022, -60.4164) (66.5951, -60.4177) (66.5879, -60.4193) (66.5807, -60.4206) knots 487 487 487 487 488 488 488 489 489 489 489
  spline S556 degree 3 poles (66.5807, -60.4206) (66.5064, -60.4346) (66.432, -60.4498) (66.3575, -60.4665) knots 489 489 489 489 490 490 490 490
  spline S557 degree 3 poles (66.3575, -60.4665) (66.346, -60.4691) (66.3346, -60.4721) (66.3232, -60.4747) knots 490 490 490 490 491 491 491 491
  spline S558 degree 3 poles (66.3232, -60.4747) (66.2531, -60.4909) (66.1831, -60.5081) (66.1131, -60.5269) (66.0979, -60.531) (66.0828, -60.5356) (66.0676, -60.5398) (66.0015, -60.5581) (65.9355, -60.5774) (65.8697, -60.5982) (65.8514, -60.604) (65.8333, -60.6103) (65.8151, -60.6163) (65.7525, -60.6368) (65.6901, -60.6581) (65.6279, -60.681) (65.6072, -60.6886) (65.5866, -60.6968) (65.5659, -60.7047) knots 491 491 491 491 492 492 492 493 493 493 494 494 494 495 495 495 496 496 496 497 497 497 497
  spline S559 degree 3 poles (65.5659, -60.7047) (65.5067, -60.7274) (65.4476, -60.7508) (65.3889, -60.7758) (65.3658, -60.7855) (65.3429, -60.7959) (65.3199, -60.806) knots 497 497 497 497 498 498 498 499 499 499 499
  spline S560 degree 3 poles (65.3199, -60.806) (65.2641, -60.8307) (65.2085, -60.8562) (65.1532, -60.8831) knots 499 499 499 499 500 500 500 500
  spline S561 degree 3 poles (65.1532, -60.8831) (65.1281, -60.8953) (65.1032, -60.9081) (65.0782, -60.9208) (65.0258, -60.9475) (64.9737, -60.9749) (64.922, -61.0036) (64.895, -61.0187) (64.8681, -61.0343) (64.8413, -61.0499) (64.7925, -61.0783) (64.744, -61.1074) (64.696, -61.1378) knots 500 500 500 500 501 501 501 502 502 502 503 503 503 504 504 504 504
  spline S562 degree 3 poles (64.696, -61.1378) (64.6671, -61.156) (64.6384, -61.1748) (64.6097, -61.1938) knots 504 504 504 504 505 505 505 505
  spline S563 degree 3 poles (64.6097, -61.1938) (64.5647, -61.2238) (64.5201, -61.2545) (64.4758, -61.2863) (64.4611, -61.2969) (64.4459, -61.3063) (64.4313, -61.3171) (64.4165, -61.328) (64.4029, -61.34) (64.3883, -61.351) (64.3658, -61.368) (64.3428, -61.3836) (64.3206, -61.401) (64.3013, -61.4162) (64.2837, -61.4331) (64.2647, -61.4485) (64.2189, -61.4858) (64.1741, -61.524) (64.13, -61.5629) (64.0955, -61.5933) (64.0611, -61.6239) (64.0277, -61.6553) (63.9839, -61.6965) (63.9415, -61.7392) (63.8994, -61.7822) (63.8682, -61.814) (63.8366, -61.8455) (63.8063, -61.8783) (63.763, -61.9253) (63.7217, -61.9742) (63.6804, -62.0232) (63.6539, -62.0545) (63.6266, -62.0848) (63.6009, -62.117) knots 505 505 505 505 506 506 506 507 507 507 508 508 508 509 509 509 510 510 510 511 511 511 512 512 512 513 513 513 514 514 514 515 515 515 516 516 516 516